Autodesk Inventor part; units mm, degrees
(part 3 of 3)
  dimension "d23" = 10.4934
  dimension "d24" = 4.2774
  dimension "d26" = 1.364
  dimension "d27" = 14.7708
  dimension "d73" = 360
  constraints: 338 point on circle, 136 centre point, 36 end point, 7 symmetric about line, 6 coincident, 6 point on line, 5 collinear, 2 equal length, 1 horizontal, 1 horizontal alignment, 1 perpendicular, 1 tangent, 1 vertical, 3126 other
  measures "d1" angle of L0 L1
  measures "d2" distance of L1.end L0.end
  measures "d12" angle of L3 L5
  measures "d15" distance from line of point (0, 0) L3
  measures "d17" distance from line of point (0, 0) L6
  measures "d18" angle of L9 L10
  measures "d19" distance from line of point (0, 0) L9
  measures "d20" angle of L12 L13
  measures "d21" distance from line of L0.start L12
  measures "d26" angle of L0 L17
  measures "d27" distance of L16.start L16.end
extrude "Extrusion1" add sketch "Sketch1" along normal blind 9.525
sketch "Sketch2" plane through (0, 9.525, 0) normal (0, 1, 0) x (1, 0, 0)
  line L0 (-6.35, 3.6662) -> (0, 7.3323)
  line L1 (0, 7.3323) -> (6.35, 3.6662)
  line L2 (6.35, 3.6662) -> (6.35, -3.6662)
  line L3 (6.35, -3.6662) -> (0, -7.3323)
  line L4 (0, -7.3323) -> (-6.35, -3.6662)
  line L5 (-6.35, -3.6662) -> (-6.35, 3.6662)
  point P0 (0, 0)
  point P1 (0, 0)
  dimension "d34" = 12.7
  constraints: 12 end point, 1 coincident, 1 vertical alignment, 13 other
  measures "d34" distance between parallel lines of L2 L5
sketch "Sketch4" plane through (0, 0, 0) normal (0, -1, 0) x (1, 0, 0)
  circle A0 centre (0, 0) radius 43.18 projected
  circle A1 centre (0, 0) radius 19.1008 construction
  line L0 (0, 0) -> (18.2308, 0) construction
  arc A2 (18.226, -0.4165) -> (18.2308, 0) centre (0, 0) ccw
  arc A3 (17.732, -0.8319) -> (18.226, -0.4165) centre (17.7962, -0.4067) ccw
  line L1 (0, 0) -> (17.5097, -2.3052) construction
  arc A4 (17.732, -0.8319) -> (16.0325, -2.1107) centre (17.5097, -2.3052) ccw
  line L2 (18.2308, 0) -> (19.1008, 0) construction
  line L3 (18.9374, -2.4932) -> (18.9042, -2.745) construction
  arc A5 (17.6096, -4.7185) -> (17.7128, -4.3149) centre (0, 0) ccw
  arc A6 (17.7128, -4.3149) -> (17.3431, -3.7859) centre (17.295, -4.2132) ccw
  arc A7 (16.0325, -2.1107) -> (17.3431, -3.7859) centre (17.5097, -2.3052) ccw
  line L4 (17.6096, -4.7185) -> (18.45, -4.9437) construction
  arc A8 (17.7128, 4.3149) -> (17.6096, 4.7185) centre (0, 0) ccw
  arc A9 (17.3431, 3.7859) -> (17.7128, 4.3149) centre (17.295, 4.2132) ccw
  arc A10 (17.3431, 3.7859) -> (16.0325, 2.1107) centre (17.5097, 2.3052) ccw
  arc A11 (16.0325, 2.1107) -> (17.732, 0.8319) centre (17.5097, 2.3052) ccw
  arc A12 (18.226, 0.4165) -> (17.732, 0.8319) centre (17.7962, 0.4067) ccw
  arc A13 (18.2308, 0) -> (18.226, 0.4165) centre (0, 0) ccw
  arc A14 (15.9925, 8.7523) -> (15.7883, 9.1154) centre (0, 0) ccw
  arc A15 (15.7723, 8.1456) -> (15.9925, 8.7523) centre (15.6153, 8.5459) ccw
  arc A16 (15.7723, 8.1456) -> (14.9399, 6.1883) centre (16.3165, 6.7585) ccw
  arc A17 (14.9399, 6.1883) -> (16.9125, 5.3929) centre (16.3165, 6.7585) ccw
  arc A18 (17.4972, 5.1196) -> (16.9125, 5.3929) centre (17.0845, 4.9988) ccw
  arc A19 (17.6096, 4.7185) -> (17.4972, 5.1196) centre (0, 0) ccw
  arc A20 (13.1823, 12.5932) -> (12.8911, 12.8911) centre (0, 0) ccw
  arc A21 (13.1266, 11.9502) -> (13.1823, 12.5932) centre (12.8714, 12.2962) ccw
  arc A22 (13.1266, 11.9502) -> (12.8292, 9.8442) centre (14.0113, 10.7512) ccw
  arc A23 (12.8292, 9.8442) -> (14.9404, 9.5864) centre (14.0113, 10.7512) ccw
  arc A24 (15.576, 9.4737) -> (14.9404, 9.5864) centre (15.2086, 9.2503) ccw
  arc A25 (15.7883, 9.1154) -> (15.576, 9.4737) centre (0, 0) ccw
  arc A26 (9.4737, 15.576) -> (9.1154, 15.7883) centre (0, 0) ccw
  arc A27 (9.5864, 14.9404) -> (9.4737, 15.576) centre (9.2503, 15.2086) ccw
  arc A28 (9.5864, 14.9404) -> (9.8442, 12.8292) centre (10.7512, 14.0113) ccw
  arc A29 (9.8442, 12.8292) -> (11.9502, 13.1266) centre (10.7512, 14.0113) ccw
  arc A30 (12.5932, 13.1823) -> (11.9502, 13.1266) centre (12.2962, 12.8714) ccw
  arc A31 (12.8911, 12.8911) -> (12.5932, 13.1823) centre (0, 0) ccw
  arc A32 (5.1196, 17.4972) -> (4.7185, 17.6096) centre (0, 0) ccw
  arc A33 (5.3929, 16.9125) -> (5.1196, 17.4972) centre (4.9988, 17.0845) ccw
  arc A34 (5.3929, 16.9125) -> (6.1883, 14.9399) centre (6.7585, 16.3165) ccw
  arc A35 (6.1883, 14.9399) -> (8.1456, 15.7723) centre (6.7585, 16.3165) ccw
  arc A36 (8.7523, 15.9925) -> (8.1456, 15.7723) centre (8.5459, 15.6153) ccw
  arc A37 (9.1154, 15.7883) -> (8.7523, 15.9925) centre (0, 0) ccw
  arc A38 (0.4165, 18.226) -> (0, 18.2308) centre (0, 0) ccw
  arc A39 (0.8319, 17.732) -> (0.4165, 18.226) centre (0.4067, 17.7962) ccw
  arc A40 (0.8319, 17.732) -> (2.1107, 16.0325) centre (2.3052, 17.5097) ccw
  arc A41 (2.1107, 16.0325) -> (3.7859, 17.3431) centre (2.3052, 17.5097) ccw
  arc A42 (4.3149, 17.7128) -> (3.7859, 17.3431) centre (4.2132, 17.295) ccw
  arc A43 (4.7185, 17.6096) -> (4.3149, 17.7128) centre (0, 0) ccw
  arc A44 (-4.3149, 17.7128) -> (-4.7185, 17.6096) centre (0, 0) ccw
  arc A45 (-3.7859, 17.3431) -> (-4.3149, 17.7128) centre (-4.2132, 17.295) ccw
  arc A46 (-3.7859, 17.3431) -> (-2.1107, 16.0325) centre (-2.3052, 17.5097) ccw
  arc A47 (-2.1107, 16.0325) -> (-0.8319, 17.732) centre (-2.3052, 17.5097) ccw
  arc A48 (-0.4165, 18.226) -> (-0.8319, 17.732) centre (-0.4067, 17.7962) ccw
  arc A49 (0, 18.2308) -> (-0.4165, 18.226) centre (0, 0) ccw
  arc A50 (-8.7523, 15.9925) -> (-9.1154, 15.7883) centre (0, 0) ccw
  arc A51 (-8.1456, 15.7723) -> (-8.7523, 15.9925) centre (-8.5459, 15.6153) ccw
  arc A52 (-8.1456, 15.7723) -> (-6.1883, 14.9399) centre (-6.7585, 16.3165) ccw
  arc A53 (-6.1883, 14.9399) -> (-5.3929, 16.9125) centre (-6.7585, 16.3165) ccw
  arc A54 (-5.1196, 17.4972) -> (-5.3929, 16.9125) centre (-4.9988, 17.0845) ccw
  arc A55 (-4.7185, 17.6096) -> (-5.1196, 17.4972) centre (0, 0) ccw
  arc A56 (-12.5932, 13.1823) -> (-12.8911, 12.8911) centre (0, 0) ccw
  arc A57 (-11.9502, 13.1266) -> (-12.5932, 13.1823) centre (-12.2962, 12.8714) ccw
  arc A58 (-11.9502, 13.1266) -> (-9.8442, 12.8292) centre (-10.7512, 14.0113) ccw
  arc A59 (-9.8442, 12.8292) -> (-9.5864, 14.9404) centre (-10.7512, 14.0113) ccw
  arc A60 (-9.4737, 15.576) -> (-9.5864, 14.9404) centre (-9.2503, 15.2086) ccw
  arc A61 (-9.1154, 15.7883) -> (-9.4737, 15.576) centre (0, 0) ccw
  arc A62 (-15.576, 9.4737) -> (-15.7883, 9.1154) centre (0, 0) ccw
  arc A63 (-14.9404, 9.5864) -> (-15.576, 9.4737) centre (-15.2086, 9.2503) ccw
  arc A64 (-14.9404, 9.5864) -> (-12.8292, 9.8442) centre (-14.0113, 10.7512) ccw
  arc A65 (-12.8292, 9.8442) -> (-13.1266, 11.9502) centre (-14.0113, 10.7512) ccw
  arc A66 (-13.1823, 12.5932) -> (-13.1266, 11.9502) centre (-12.8714, 12.2962) ccw
  arc A67 (-12.8911, 12.8911) -> (-13.1823, 12.5932) centre (0, 0) ccw
  arc A68 (-17.4972, 5.1196) -> (-17.6096, 4.7185) centre (0, 0) ccw
  arc A69 (-16.9125, 5.3929) -> (-17.4972, 5.1196) centre (-17.0845, 4.9988) ccw
  arc A70 (-16.9125, 5.3929) -> (-14.9399, 6.1883) centre (-16.3165, 6.7585) ccw
  arc A71 (-14.9399, 6.1883) -> (-15.7723, 8.1456) centre (-16.3165, 6.7585) ccw
  arc A72 (-15.9925, 8.7523) -> (-15.7723, 8.1456) centre (-15.6153, 8.5459) ccw
  arc A73 (-15.7883, 9.1154) -> (-15.9925, 8.7523) centre (0, 0) ccw
  arc A74 (-18.226, 0.4165) -> (-18.2308, 0) centre (0, 0) ccw
  arc A75 (-17.732, 0.8319) -> (-18.226, 0.4165) centre (-17.7962, 0.4067) ccw
  arc A76 (-17.732, 0.8319) -> (-16.0325, 2.1107) centre (-17.5097, 2.3052) ccw
  arc A77 (-16.0325, 2.1107) -> (-17.3431, 3.7859) centre (-17.5097, 2.3052) ccw
  arc A78 (-17.7128, 4.3149) -> (-17.3431, 3.7859) centre (-17.295, 4.2132) ccw
  arc A79 (-17.6096, 4.7185) -> (-17.7128, 4.3149) centre (0, 0) ccw
  arc A80 (-17.7128, -4.3149) -> (-17.6096, -4.7185) centre (0, 0) ccw
  arc A81 (-17.3431, -3.7859) -> (-17.7128, -4.3149) centre (-17.295, -4.2132) ccw
  arc A82 (-17.3431, -3.7859) -> (-16.0325, -2.1107) centre (-17.5097, -2.3052) ccw
  arc A83 (-16.0325, -2.1107) -> (-17.732, -0.8319) centre (-17.5097, -2.3052) ccw
  arc A84 (-18.226, -0.4165) -> (-17.732, -0.8319) centre (-17.7962, -0.4067) ccw
  arc A85 (-18.2308, 0) -> (-18.226, -0.4165) centre (0, 0) ccw
  arc A86 (-15.9925, -8.7523) -> (-15.7883, -9.1154) centre (0, 0) ccw
  arc A87 (-15.7723, -8.1456) -> (-15.9925, -8.7523) centre (-15.6153, -8.5459) ccw
  arc A88 (-15.7723, -8.1456) -> (-14.9399, -6.1883) centre (-16.3165, -6.7585) ccw
  arc A89 (-14.9399, -6.1883) -> (-16.9125, -5.3929) centre (-16.3165, -6.7585) ccw
  arc A90 (-17.4972, -5.1196) -> (-16.9125, -5.3929) centre (-17.0845, -4.9988) ccw
  arc A91 (-17.6096, -4.7185) -> (-17.4972, -5.1196) centre (0, 0) ccw
  arc A92 (-13.1823, -12.5932) -> (-12.8911, -12.8911) centre (0, 0) ccw
  arc A93 (-13.1266, -11.9502) -> (-13.1823, -12.5932) centre (-12.8714, -12.2962) ccw
  arc A94 (-13.1266, -11.9502) -> (-12.8292, -9.8442) centre (-14.0113, -10.7512) ccw
  arc A95 (-12.8292, -9.8442) -> (-14.9404, -9.5864) centre (-14.0113, -10.7512) ccw
  arc A96 (-15.576, -9.4737) -> (-14.9404, -9.5864) centre (-15.2086, -9.2503) ccw
  arc A97 (-15.7883, -9.1154) -> (-15.576, -9.4737) centre (0, 0) ccw
  arc A98 (-9.4737, -15.576) -> (-9.1154, -15.7883) centre (0, 0) ccw
  arc A99 (-9.5864, -14.9404) -> (-9.4737, -15.576) centre (-9.2503, -15.2086) ccw
  arc A100 (-9.5864, -14.9404) -> (-9.8442, -12.8292) centre (-10.7512, -14.0113) ccw
  arc A101 (-9.8442, -12.8292) -> (-11.9502, -13.1266) centre (-10.7512, -14.0113) ccw
  arc A102 (-12.5932, -13.1823) -> (-11.9502, -13.1266) centre (-12.2962, -12.8714) ccw
  arc A103 (-12.8911, -12.8911) -> (-12.5932, -13.1823) centre (0, 0) ccw
  arc A104 (-5.1196, -17.4972) -> (-4.7185, -17.6096) centre (0, 0) ccw
  arc A105 (-5.3929, -16.9125) -> (-5.1196, -17.4972) centre (-4.9988, -17.0845) ccw
  arc A106 (-5.3929, -16.9125) -> (-6.1883, -14.9399) centre (-6.7585, -16.3165) ccw
  arc A107 (-6.1883, -14.9399) -> (-8.1456, -15.7723) centre (-6.7585, -16.3165) ccw
  arc A108 (-8.7523, -15.9925) -> (-8.1456, -15.7723) centre (-8.5459, -15.6153) ccw
  arc A109 (-9.1154, -15.7883) -> (-8.7523, -15.9925) centre (0, 0) ccw
  arc A110 (-0.4165, -18.226) -> (0, -18.2308) centre (0, 0) ccw
  arc A111 (-0.8319, -17.732) -> (-0.4165, -18.226) centre (-0.4067, -17.7962) ccw
  arc A112 (-0.8319, -17.732) -> (-2.1107, -16.0325) centre (-2.3052, -17.5097) ccw
  arc A113 (-2.1107, -16.0325) -> (-3.7859, -17.3431) centre (-2.3052, -17.5097) ccw
  arc A114 (-4.3149, -17.7128) -> (-3.7859, -17.3431) centre (-4.2132, -17.295) ccw
  arc A115 (-4.7185, -17.6096) -> (-4.3149, -17.7128) centre (0, 0) ccw
  arc A116 (4.3149, -17.7128) -> (4.7185, -17.6096) centre (0, 0) ccw
  arc A117 (3.7859, -17.3431) -> (4.3149, -17.7128) centre (4.2132, -17.295) ccw
  arc A118 (3.7859, -17.3431) -> (2.1107, -16.0325) centre (2.3052, -17.5097) ccw
  arc A119 (2.1107, -16.0325) -> (0.8319, -17.732) centre (2.3052, -17.5097) ccw
  arc A120 (0.4165, -18.226) -> (0.8319, -17.732) centre (0.4067, -17.7962) ccw
  arc A121 (0, -18.2308) -> (0.4165, -18.226) centre (0, 0) ccw
  arc A122 (8.7523, -15.9925) -> (9.1154, -15.7883) centre (0, 0) ccw
  arc A123 (8.1456, -15.7723) -> (8.7523, -15.9925) centre (8.5459, -15.6153) ccw
  arc A124 (8.1456, -15.7723) -> (6.1883, -14.9399) centre (6.7585, -16.3165) ccw
  arc A125 (6.1883, -14.9399) -> (5.3929, -16.9125) centre (6.7585, -16.3165) ccw
  arc A126 (5.1196, -17.4972) -> (5.3929, -16.9125) centre (4.9988, -17.0845) ccw
  arc A127 (4.7185, -17.6096) -> (5.1196, -17.4972) centre (0, 0) ccw
  arc A128 (12.5932, -13.1823) -> (12.8911, -12.8911) centre (0, 0) ccw
  arc A129 (11.9502, -13.1266) -> (12.5932, -13.1823) centre (12.2962, -12.8714) ccw
  arc A130 (11.9502, -13.1266) -> (9.8442, -12.8292) centre (10.7512, -14.0113) ccw
  arc A131 (9.8442, -12.8292) -> (9.5864, -14.9404) centre (10.7512, -14.0113) ccw
  arc A132 (9.4737, -15.576) -> (9.5864, -14.9404) centre (9.2503, -15.2086) ccw
  arc A133 (9.1154, -15.7883) -> (9.4737, -15.576) centre (0, 0) ccw
  arc A134 (15.576, -9.4737) -> (15.7883, -9.1154) centre (0, 0) ccw
  arc A135 (14.9404, -9.5864) -> (15.576, -9.4737) centre (15.2086, -9.2503) ccw
  arc A136 (14.9404, -9.5864) -> (12.8292, -9.8442) centre (14.0113, -10.7512) ccw
  arc A137 (12.8292, -9.8442) -> (13.1266, -11.9502) centre (14.0113, -10.7512) ccw
  arc A138 (13.1823, -12.5932) -> (13.1266, -11.9502) centre (12.8714, -12.2962) ccw
  arc A139 (12.8911, -12.8911) -> (13.1823, -12.5932) centre (0, 0) ccw
  arc A140 (17.4972, -5.1196) -> (17.6096, -4.7185) centre (0, 0) ccw
  arc A141 (16.9125, -5.3929) -> (17.4972, -5.1196) centre (17.0845, -4.9988) ccw
  arc A142 (16.9125, -5.3929) -> (14.9399, -6.1883) centre (16.3165, -6.7585) ccw
  arc A143 (14.9399, -6.1883) -> (15.7723, -8.1456) centre (16.3165, -6.7585) ccw
  arc A144 (15.9925, -8.7523) -> (15.7723, -8.1456) centre (15.6153, -8.5459) ccw
  arc A145 (15.7883, -9.1154) -> (15.9925, -8.7523) centre (0, 0) ccw
  point P0 (18.2308, 0)
  point P1 (17.6096, 4.7185)
  point P2 (15.7883, 9.1154)
  point P3 (9.1154, 15.7883)
  point P4 (4.7185, 17.6096)
  point P5 (0, 18.2308)
  point P6 (-4.7185, 17.6096)
  point P7 (-9.1154, 15.7883)
  point P8 (-12.8911, 12.8911)
  point P9 (-15.7883, 9.1154)
  point P10 (-17.6096, 4.7185)
  point P11 (-18.2308, 0)
  point P12 (-17.6096, -4.7185)
  point P13 (-15.7883, -9.1154)
  point P14 (-12.8911, -12.8911)
  point P15 (-9.1154, -15.7883)
  point P16 (-4.7185, -17.6096)
  point P17 (0, -18.2308)
  point P18 (4.7185, -17.6096)
  point P19 (9.1154, -15.7883)
  point P20 (12.8911, -12.8911)
  point P21 (15.7883, -9.1154)
  dimension "d41" = 38.2016
  dimension "d43" = 0.43
  dimension "d44" = 1.49
  dimension "d45" = 0.87
  dimension "d46" = 2.93
  dimension "d47" = 0.254
  dimension "d48" = 7.5
  dimension "d55" = 360
  constraints: 290 point on circle, 145 centre point, 10 end point, 5 symmetric about line, 3 tangent, 2 horizontal, 2 point on line, 1 coincident, 1 concentric, 412 other
  measures "d41" diameter of A1
  measures "d43" radius of A3
  measures "d44" radius of A4
  measures "d45" distance of L0.end L2.end
  measures "d46" distance from line of A4.end L3
  measures "d47" distance of L3.start L3.end
  measures "d48" angle of L0 L1
extrude "Extrusion4" add sketch "Sketch4" along normal blind 10 contours A3 A4 A7 A6 A5 A140 A141 A142 A143 A144 A145 A134 A135 A136 A137 A138 A139 A128 A129 A130 A131 A132 A133 A122 A123 A124 A125 A126 A127 A116 A117 A118 A119 A120 A121 A110 A111 A112 A113 A114 A115 A104 A105 A106 A107 A108 A109 A98 A99 A100 A101 A102 A103 A92 A93 A94 A95 A96 A97 A86 A87 A88 A89 A90 A91 A80 A81 A82 A83 A84 A85 A74 A75 A76 A77 A78 A79 A68 A69 A70 A71 A72 A73 A62 A63 A64 A65 A66 A67 A56 A57 A58 A59 A60 A61 A50 A51 A52 A53 A54 A55 A44 A45 A46 A47 A48 A49 A38 A39 A40 A41 A42 A43 A32 A33 A34 A35 A36 A37 A26 A27 A28 A29 A30 A31 A20 A21 A22 A23 A24 A25 A14 A15 A16 A17 A18 A19 A8 A9 A10 A11 A12 A13 A2
sketch "Sketch5" plane through (0, -10, 0) normal (0, -1, 0) x (1, 0, 0)
  circle A0 centre (0, 0) radius 19.1008
  dimension "d59" = 38.2016
  constraints: 1 centre point, 1 coincident
  measures "d59" diameter of A0
extrude "Extrusion5" add sketch "Sketch5" along normal blind 0.635
extrude "Extrusion7" cut sketch "Sketch2" along normal through all both and the other way through all
sketch "Sketch6" plane through (0, 9.525, 0) normal (0, 1, 0) x (1, 0, 0)
  circle A0 centre (0, 0) radius 8.89
  line L0 (-6.35, 3.6662) -> (0, 7.3323)
  line L1 (0, 7.3323) -> (6.35, 3.6662)
  line L2 (6.35, 3.6662) -> (6.35, -3.6662)
  line L3 (6.35, -3.6662) -> (0, -7.3323)
  line L4 (0, -7.3323) -> (-6.35, -3.6662)
  line L5 (-6.35, -3.6662) -> (-6.35, 3.6662)
  dimension "d66" = 17.78
  dimension "d67" = 12.7
  dimension "d68" = 3.6662
  constraints: 12 end point, 2 coincident, 1 centre point, 13 other
  measures "d66" diameter of A0
  measures "d67" distance between parallel lines of L2 L5
  measures "d68" vertical distance of A0.centre L4.end
extrude "Extrusion8" add sketch "Sketch6" along normal blind 2.794
extrude "Extrusion9" cut sketch "Sketch1" along normal through all contours A3 S2 S3 A7 A4 S1 S0 | S5 S6 A8 A9 S7 S4 A3 | S9 S10 A10 A11 S11 S8 A3 | S13 S14 A12 A13 S15 S12 A3 | S17 S18 A14 A15 S19 S16 A3 | S21 S22 A16 A17 S23 S20 A3 | S25 S26 A18 A19 S27 S24 A3 | S29 S30 A20 A21 S31 S28 A3 | S33 S34 A22 A23 S35 S32 A3 | S37 S38 A24 A25 S39 S36 A3 | S41 S42 A26 A27 S43 S40 A3 | S45 S46 A28 A29 S47 S44 A3 | S49 S50 A30 A31 S51 S48 A3 | S53 S54 A32 A33 S55 S52 A3 | A3 S213 S214 A112 A113 S215 S212 | S57 S58 A34 A35 S59 S56 A3 | A3 S209 S210 A110 A111 S211 S208 | S61 S62 A36 A37 S63 S60 A3 | A3 S205 S206 A108 A109 S207 S204 | S65 S66 A38 A39 S67 S64 A3 | A3 S201 S202 A106 A107 S203 S200 | S69 S70 A40 A41 S71 S68 A3 | A3 S197 S198 A104 A105 S199 S196 | S73 S74 A42 A43 S75 S72 A3 | A3 S193 S194 A102 A103 S195 S192 | S77 S78 A44 A45 S79 S76 A3 | A3 S189 S190 A100 A101 S191 S188 | S81 S82 A46 A47 S83 S80 A3 | A3 S185 S186 A98 A99 S187 S184 | S85 S86 A48 A49 S87 S84 A3 | A3 S181 S182 A96 A97 S183 S180 | S89 S90 A50 A51 S91 S88 A3 | A3 S177 S178 A94 A95 S179 S176 | S93 S94 A52 A53 S95 S92 A3 | A3 S173 S174 A92 A93 S175 S172 | S97 S98 A54 A55 S99 S96 A3 | A3 S169 S170 A90 A91 S171 S168 | S101 S102 A56 A57 S103 S100 A3 | A3 S165 S166 A88 A89 S167 S164 | S105 S106 A58 A59 S107 S104 A3 | A3 S161 S162 A86 A87 S163 S160 | S109 S110 A60 A61 S111 S108 A3 | A3 S157 S158 A84 A85 S159 S156 | S113 S114 A62 A63 S115 S112 A3 | A3 S153 S154 A82 A83 S155 S152 | S117 S118 A64 A65 S119 S116 A3 | A3 S149 S150 A80 A81 S151 S148 | S121 S122 A66 A67 S123 S120 A3 | A3 S145 S146 A78 A79 S147 S144 | S125 S126 A68 A69 S127 S124 A3 | A3 S141 S142 A76 A77 S143 S140 | S129 S130 A70 A71 S131 S128 A3 | A3 S137 S138 A74 A75 S139 S136 | S133 S134 A72 A73 S135 S132 A3
extrude "Extrusion10" cut sketch "Sketch1" along normal blind 25.4 contours A3 S261 S262 A136 A137 S263 S260 | A3 S257 S258 A134 A135 S259 S256 | A3 S253 S254 A132 A133 S255 S252 | A3 S249 S250 A130 A131 S251 S248 | A3 S245 S246 A128 A129 S247 S244 | A3 S241 S242 A126 A127 S243 S240 | A3 S237 S238 A124 A125 S239 S236 | A3 S233 S234 A122 A123 S235 S232 | A3 S229 S230 A120 A121 S231 S228 | A3 S225 S226 A118 A119 S227 S224 | A3 S221 S222 A116 A117 S223 S220 | A3 S217 S218 A114 A115 S219 S216
body "Solid1"
